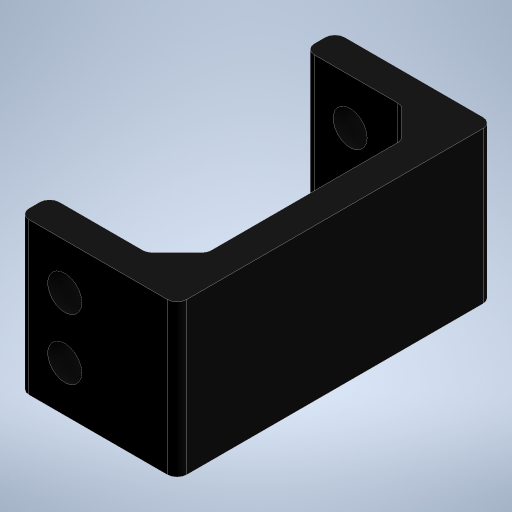
# Autodesk Inventor part: finger_rig
Saved by Autodesk Inventor 2024.2 (Build 282272000, 272)
## iProperties
Created: 2024-01-09
Part Number: finger_rig
Material: PLA
Document SubType Name: Modeling
Designer: Konrad
Density: 1 g/cm^3
Appearance: PLA
Author: Konrad
Autodesk Inventor part; units mm, degrees
ref_plane "YZ Plane" through (0, 0, 0) normal (1, 0, 0) x (0, 1, 0)
ref_plane "XZ Plane" through (0, 0, 0) normal (0, 1, 0) x (-1, 0, 0)
ref_plane "XY Plane" through (0, 0, 0) normal (0, 0, 1) x (1, 0, 0)
sketch "Szkic1" plane through (0, 0, 0) normal (0, 0, 1) x (1, 0, 0)
  line L0 (0, 0) -> (21, 0)
  line L1 (21, 0) -> (21, 25)
  line L2 (21, 25) -> (0, 25)
  line L3 (0, 25) -> (0, 0)
  line L4 (21, 25) -> (26, 25)
  line L5 (26, 25) -> (26, 0)
  line L6 (26, 0) -> (21, 0)
  line L7 (21, 0) -> (21, 25)
  line L8 (0, 12.5) -> (26, 12.5) construction
  circle A0 centre (7.5, 17.5) radius 2.8
  circle A1 centre (7.5, 7.5) radius 2.8
  dimension "d0" = 21
  dimension "d1" = 25
  dimension "d2" = 5
  dimension "d4" = 7.5
  dimension "d5" = 5.6
  dimension "d13" = 10
  constraints: 18 end point, 4 parallel, 2 centre point, 2 horizontal, 2 midpoint, 2 perpendicular, 1 equal radius, 1 symmetric about line, 1 other
  measures "d0" distance of L2.end L1.end
  measures "d1" distance of L1.end L0.end
  measures "d2" distance of L5.end L6.end
  measures "d4" distance from line of L3 A0.centre
  measures "d5" diameter of A1
  measures "d13" distance of A1.centre A0.centre
extrude "Wyciągnięcie proste1" add sketch "Szkic1" along normal mid plane 52
extrude "Wyciągnięcie proste2" cut sketch "Szkic1" along normal mid plane 42 contours L3 L2 L1 L0
chamfer "Faza1" distance 5 angle 45 2 edges at (21, 12.5, 21) (21, 12.5, -21)
fillet "Zaokrąglenie1" radius 1.6 10 edges at (0, 12.5, 26) (0, 12.5, 21) (26, 12.5, 26) (26, 12.5, -26) (0, 12.5, -26) (0, 12.5, -21) (16, 12.5, 21) (21, 12.5, 16) (21, 12.5, -16) (16, 12.5, -21)
